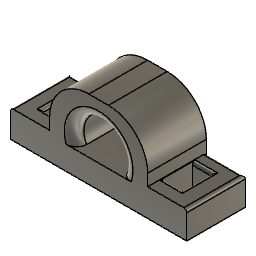
palm guide (Autodesk Fusion 360 design; units mm, degrees)
Autodesk Fusion 360 part; units mm, degrees
note: some values were not read from the file. Chosen so that the rebuilt part matches the saved one: which face or edge a step refers to; which pieces of a blend or face edit are solid.
sketch "Sketch1" plane through (0, 0, 0) normal (0, 0, 1) x (1, 0, 0)
  line L0 (0, 0) -> (5, 0)
  line L1 (5, 0) -> (5, 4)
  line L2 (5, 4) -> (0, 4)
  line L3 (0, 4) -> (0, 0)
  dimension "d1" = 5
  dimension "d2" = 4
  constraint horizontal L0
  constraint vertical L1
  constraint horizontal L2
  constraint vertical L3
  constraint coincident L0.start L3.end
  measures "d1" distance of L0.start L0.end
  measures "d2" distance of L0.start L2.end
extrude "Extrude1" add sketch "Sketch1" along normal blind 4
sketch "Sketch2" plane through (0, 0, 0) normal (0, -1, 0) x (1, 0, 0)
  line L0 (0, 0) -> (5, 0)
  line L1 (5, 0) -> (5, 4)
  line L2 (5, 4) -> (0, 4)
  line L3 (0, 4) -> (0, 0)
  circle A0 centre (2.5, 4) radius 4
  line L4 (3.6225, 1.2) -> (1.3775, 1.2)
  arc A1 (3.6225, 1.2) -> (1.3775, 1.2) centre (2.5, 1.75) ccw
  dimension "d5" = 2.5
  dimension "d6" = 1.75
  dimension "d7" = 1.2
  dimension "d30" = 2.5
  constraint midpoint L2 A0.centre
  constraint tangent L0 A0
  constraint perpendicular L1 L4
  measures "d5" diameter of A1
  measures "d6" distance of L0 A1.centre
  measures "d7" distance of L0 L4
  measures "d30" distance of L3 A1.centre
extrude "Extrude2" cut sketch "Sketch2" against normal blind 7 contours L4 A1
fillet "Fillet1" radius 0.75 2 edges at (2.5, 0, 3) (2.5, 4, 3)
fillet "Fillet2" radius 0.5 2 edges at (2.5, 0, 1.2) (2.5, 4, 1.2)
fillet "Fillet3" radius 2 2 edges at (5, 2, 4) (0, 2, 4)
sketch "Sketch3" plane through (0, 0, 0) normal (0, 0, -1) x (1, 0, 0)
  line L0 (0, 0) -> (0, -4)
  line L1 (0, -4) -> (5, -4)
  line L2 (5, -4) -> (5, 0)
  line L3 (5, 0) -> (0, 0)
  line L4 (0, 0) -> (-2, 0)
  line L5 (-2, 0) -> (-2, -4)
  line L6 (-2, -4) -> (0, -4)
  line L7 (0, -4) -> (0, 0)
  line L8 (5, 0) -> (7, 0)
  line L9 (7, 0) -> (7, -4)
  line L10 (7, -4) -> (5, -4)
  line L11 (5, -4) -> (5, 0)
  line L12 (-1.1104, -3.25) -> (-0.1104, -3.25)
  line L13 (-0.1104, -3.25) -> (-0.1104, -1.75)
  line L14 (-0.1104, -1.75) -> (-1.1104, -1.75)
  line L15 (-1.1104, -1.75) -> (-1.1104, -3.25)
  line L16 (6.0316, -3.25) -> (5.0316, -3.25)
  line L17 (5.0316, -3.25) -> (5.0316, -1.75)
  line L18 (5.0316, -1.75) -> (6.0316, -1.75)
  line L19 (6.0316, -1.75) -> (6.0316, -3.25)
  dimension "d31" = 4
  dimension "d32" = 4
  dimension "d33" = 2
  dimension "d34" = 2
  dimension "d35" = 1
  dimension "d36" = 1.5
  dimension "d37" = 0.75
  dimension "d38" = 1
  dimension "d39" = 1.5
  dimension "d40" = 0.75
  constraint horizontal L4
  constraint vertical L5
  constraint horizontal L6
  constraint vertical L7
  constraint coincident L0.start L3.end
  constraint horizontal L8
  constraint vertical L9
  constraint horizontal L10
  constraint vertical L11
  constraint coincident L2.end L3.start
  constraint horizontal L12
  constraint vertical L13
  constraint horizontal L14
  constraint vertical L15
  constraint horizontal L16
  constraint vertical L17
  constraint horizontal L18
  constraint vertical L19
  measures "d31" distance of L4.end L5.end
  measures "d32" distance of L8.end L9.end
  measures "d33" distance of L2.end L8.end
  measures "d34" distance of L0.start L4.end
  measures "d35" distance of L12.start L12.end
  measures "d36" distance of L12.start L14.end
  measures "d37" distance of L6 L12
  measures "d38" distance of L16.start L16.end
  measures "d39" distance of L16.start L18.end
  measures "d40" distance of L10 L16
extrude "Extrude3" add sketch "Sketch3" against normal blind 1.4 contours L0 L4 L5 L6 L7 | L2 L8 L9 L10 L11
sketch "Sketch6" plane through (0, 0, 0) normal (0, -1, 0) x (1, 0, 0)
  arc A0 (2, 4) -> (0, 2) centre (2, 2) ccw
  line L0 (0, 2) -> (0, 1.4)
  line L1 (0, 1.4) -> (-2, 1.4)
  line L2 (-2, 1.4) -> (-2, 0)
  line L3 (-2, 0) -> (7, 0)
  line L4 (7, 0) -> (7, 1.4)
  line L5 (7, 1.4) -> (5, 1.4)
  line L6 (5, 1.4) -> (5, 2)
  arc A1 (5, 2) -> (3, 4) centre (3, 2) ccw
  line L7 (3, 4) -> (2, 4)
  arc A2 (4.2022, 0.7) -> (0.7978, 0.7) centre (2.5, 1.75) ccw
  line L8 (4.2022, 0.7) -> (0.7978, 0.7)
  line L9 (-2.7359, -1.8675) -> (8.734, -1.8675)
  line L10 (8.734, -1.8675) -> (8.734, 4.3723)
  line L11 (8.734, 4.3723) -> (-2.7359, 4.3723)
  line L12 (-2.7359, 4.3723) -> (-2.7359, -1.8675)
  constraint horizontal L9
  constraint vertical L10
  constraint horizontal L11
  constraint vertical L12
extrude "Extrude7" cut sketch "Sketch6" against normal blind 1 contours A0 L0 L1 L2 L3 L4 L5 L6 A1 L7 | A2 L8 | L9 L10 L11 L12
fillet "Fillet4" radius 0.15 10 edges at (-1, 4, 1.4) (6, 4, 1.4) (7, 2.5, 1.4) (-2, 2.5, 1.4) (-1.1104, 2.5, 1.4) (-0.6104, 1.75, 1.4) (-0.6104, 3.25, 1.4) (5.5316, 3.25, 1.4) (6.0316, 2.5, 1.4) (5.5316, 1.75, 1.4)
fillet "Fillet5" radius 0.5 1 edges at (2.5, 1, 3)
